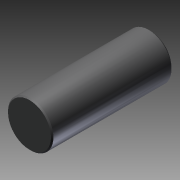
# Autodesk Inventor part: D-358
Saved by Autodesk Inventor 2011 SP1 (Build 150282100, 282)
## iProperties
Created: 2016-10-01
Part Number: D-358
Catalog Web Link: www.cadenas.de
Description: Pin-Original Line - Standard Air Cylinders
Vendor: BIMBA
Document SubType Name: Modeling
Designer: psAdmin
Manufacturer: BIMBA
Mass: 1.80712 g
Surface Area: 8.91685 cm^2
Volume: 1.80712 cm^3
Density: 1 g/cm^3
Category: PARTsolutions
Company: BIMBA
Title: D-358
Author: Cadenas PARTsolutions
Comments: Original Line - Standard Air Cylinders
PSOL_IDENT_0: {$CADENAS_DATA\23d-libs\bimba\bimba\bimba_imperial\bimba_full_line\original_line_cylinders\standard_
PSOL_IDENT_1: air_cylinders\pin.prj},149 {VTYP=3D},{NB=D-358},{LINA=D-358},{NN=Pin},{DATE=22.09.2016 13:52:24},{GE
PSOL_IDENT_2: OMDATE=15.02.2011 00:00:00},{VERSION=},{LINEID=30},{LINESUBID=-1},{WBVAR=}  {NB=D-358},{LINA=D-358},
PSOL_IDENT_3: {KT=DUMMY},{PN=D-358},{DIA=0.37500},{L=1.0000}
NN: Pin
NT: Original Line - Standard Air Cylinders
NB: D-358
NBSYN: $PN.
LINA: D-358
PN: D-358
DIA: 0.37500
L: 1.0000
SUPPLIER: BIMBA
ARTICLENO: D-358
BOMINFO: D-358
CREATOR: CADENAS GmbH
Autodesk Inventor part; units mm, degrees
ref_plane "YZ Plane" through (0, 0, 0) normal (1, 0, 0) x (0, 1, 0)
ref_plane "XZ Plane" through (0, 0, 0) normal (0, 1, 0) x (-1, 0, 0)
ref_plane "XY Plane" through (0, 0, 0) normal (0, 0, 1) x (1, 0, 0)
sketch "Sketch_1" plane through (0, 0, 0) normal (1, 0, 0) x (0, 1, 0)
  line L0 (0, -12.7) -> (0, 12.7)
  line L1 (0, 12.7) -> (4.5111, 12.7)
  line L2 (4.5111, 12.7) -> (4.7625, 12.4486)
  line L3 (4.7625, 12.4486) -> (4.7625, -12.3444)
  line L4 (4.7625, -12.3444) -> (4.4069, -12.7)
  line L5 (4.4069, -12.7) -> (0, -12.7)
  line L6 (0, -12.7) -> (0, 12.7)
  constraints: 14 end point
revolve "Revolution1" add sketch "Sketch_1" angle 360 about axis through (0, 0, -12.7) along (0, 0, -1)
ref_plane "dia1_XY" through (-4.7625, 0, 0) normal (0, 0, 1) x (1, 0, 0)
ref_plane "dia1_YZ" through (-4.7625, 0, 0) normal (1, 0, 0) x (0, 1, 0)
ref_plane "dia1_ZX" through (-4.7625, 0, 0) normal (0, 1, 0) x (0, 0, 1)
ref_plane "dia2_XY" through (4.7625, 0, 0) normal (0, 0, 1) x (1, 0, 0)
ref_plane "dia2_YZ" through (4.7625, 0, 0) normal (1, 0, 0) x (0, 1, 0)
ref_plane "dia2_ZX" through (4.7625, 0, 0) normal (0, 1, 0) x (0, 0, 1)
ref_plane "pin_XY" through (0, 0, 0) normal (0, 0, 1) x (1, 0, 0)
ref_plane "pin_YZ" through (0, 0, 0) normal (1, 0, 0) x (0, 1, 0)
ref_plane "pin_ZX" through (0, 0, 0) normal (0, 1, 0) x (0, 0, 1)
ref_plane "pin1_XY" through (0, 0, 12.7) normal (1, 0, 0) x (0, 0, -1)
ref_plane "pin1_YZ" through (0, 0, 12.7) normal (0, 0, -1) x (0, 1, 0)
ref_plane "pin1_ZX" through (0, 0, 12.7) normal (0, 1, 0) x (1, 0, 0)
ref_plane "pin2_XY" through (0, 0, -12.7) normal (1, 0, 0) x (0, 0, -1)
ref_plane "pin2_YZ" through (0, 0, -12.7) normal (0, 0, -1) x (0, 1, 0)
ref_plane "pin2_ZX" through (0, 0, -12.7) normal (0, 1, 0) x (1, 0, 0)
body "Solid1"
